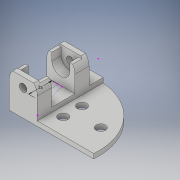
# Autodesk Inventor part: beta_plate
Saved by Autodesk Inventor 2018 (Build 220112000, 112)
## iProperties
Created: 2017-10-04
Part Number: beta_plate
Material: Generic
Document SubType Name: Modeling
Designer: rheal
Density: 1 g/cm^3
Appearance: Default
Author: rheal
Autodesk Inventor part; units mm, degrees
ref_plane "Work Plane12" through (0, 0, 0) normal (0, 1, 0) x (1, 0, 0)
sketch "Sketch2" plane through (0, 0, 0) normal (0, 1, 0) x (1, 0, 0)
  line L0 (-10, -65) -> (-10, -85)
  line L1 (-10, -85) -> (20, -85)
  line L2 (-10, -50) -> (-10, -15)
  line L3 (17.5697, -20.0796) -> (74.4447, -85.0796) construction
  line L4 (80.25, -80) -> (80.25, -36.3042) construction
  line L5 (-10, -65) -> (-10, -50)
  arc A0 (80.25, -80) -> (23.375, -15) centre (15.252, -79.4904) ccw projected
  line L6 (20, -85) -> (20, -15)
  line L7 (20, -85) -> (90, -85) construction
  line L8 (20, -15) -> (-10, -15)
  point P0 (0, -80)
  point P1 (0, 0)
  dimension "d13" = 30
  dimension "d14" = 20
  dimension "d15" = 35
  dimension "d98" = 70
  dimension "d99" = 90
  constraints: 16 end point, 3 vertical, 1 horizontal, 1 perpendicular, 1 other
  measures "d13" distance of L1.end L0.end
  measures "d14" distance of L0.end L0.start
  measures "d15" distance of L2.start L2.end
  measures "d98" distance of L1.end L6.end
  measures "d99" angle of L7 L6
extrude "Extrusion2" add sketch "Sketch2" along normal blind 5
ref_plane "Work Plane7" through (0, 5, 0) normal (0, 1, 0) x (1, 0, 0)
ref_plane "Work Plane6" through (0, 5, 0) normal (0, 1, 0) x (1, 0, 0)
sketch "Sketch7" plane through (0, 5, 0) normal (0, 1, 0) x (1, 0, 0)
  line L0 (-2.5, -32.5) -> (7.5, -32.5) projected
  line L1 (2.5, -32.5) -> (15, -75.625) construction
  line L2 (15, -85) -> (15, -65) projected
  line L3 (-2.5, -45) -> (7.5, -45) projected
  line L4 (2.5, -45) -> (2.5, -70) construction
  line L5 (2.5, -57.5) -> (-13.1217, -57.5) construction
  point P0 (0, 0)
  point P1 (20, -85)
  dimension "d54" = 25
  constraints: 6 end point, 3 midpoint, 1 horizontal, 1 vertical, 2 other
  measures "d54" distance of L4.start L4.end
ref_plane "Work Plane8" through (-2.5, 5, 45) normal (0, 0, 1) x (1, 0, 0)
sketch "Sketch8" plane through (-2.5, 5, 45) normal (0, 0, 1) x (1, 0, 0)
  line L0 (-7.5, 0) -> (22.5, 0) projected
  arc A0 (22.5, 18) -> (-7.5, 18) centre (7.5, 18) ccw
  line L1 (-7.5, 18) -> (-7.5, 0)
  line L2 (22.5, 18) -> (22.5, 0)
  point P0 (2.5, -5)
  dimension "d100" = 30
  constraints: 4 end point, 2 point on circle, 1 centre point, 1 parallel, 1 vertical
  measures "d100" diameter of A0
extrude "Extrusion7" add sketch "Sketch8" against normal blind 15
ref_plane "Work Plane9" through (-2.5, 5, 45) normal (0, 0, 1) x (1, 0, 0)
sketch "Sketch9" plane through (-2.5, 5, 45) normal (0, 0, 1) x (1, 0, 0)
  arc A0 (-2, 18) -> (17, 18) centre (7.5, 18) ccw
  line L0 (-2, 18) -> (-2, 26.124)
  line L1 (17, 18) -> (17, 26.124)
  line L2 (22.5, 0) -> (-7.5, 0) construction
  line L3 (7.5, 0) -> (7.5, 18) construction
  arc A1 (22.5, 18) -> (-7.5, 18) centre (7.5, 18) ccw construction
  line L4 (17, 26.124) -> (20.1095, 26.124)
  line L5 (-2, 26.124) -> (-5.1095, 26.124)
  arc A2 (20.1095, 26.124) -> (-5.1095, 26.124) centre (7.5, 18) ccw
  point P0 (2.5, -5)
  dimension "d47" = 19
  constraints: 10 end point, 6 point on circle, 2 centre point, 1 concentric, 1 horizontal, 1 midpoint, 1 point on line
  measures "d47" diameter of A0
extrude "Extrusion8" cut sketch "Sketch9" against normal blind 10
ref_plane "Work Plane10" through (2.5, 23, 30) normal (0, 0, -1) x (-1, 0, 0)
sketch "Sketch10" plane through (2.5, 23, 30) normal (0, 0, -1) x (-1, 0, 0)
  line L0 (-5, 0) -> (5, 0) projected
  arc A0 (-12, 0) -> (7, 0) centre (-2.5, 0) ccw projected
  circle A1 centre (-2.5, 0) radius 4
  point P0 (2.5, -23)
  dimension "d103" = 8
  constraints: 1 centre point, 1 coincident
  measures "d103" diameter of A1
extrude "Extrusion9" cut sketch "Sketch10" against normal blind 5
ref_plane "Work Plane2" through (2.5, 5, 57.5) normal (0, 0, 1) x (1, 0, 0)
mirror "Mirror2" about plane through (2.5, 5, 57.5) normal (0, 0, 1) of "Extrusion7", "Extrusion8", "Extrusion9"
ref_plane "Work Plane11" through (2.5, 23, 85) normal (0, 0, 1) x (1, 0, 0)
sketch "Sketch11" plane through (2.5, 23, 85) normal (0, 0, 1) x (1, 0, 0)
  line L0 (-12.5, 20) -> (17.5, 20)
  line L1 (17.5, 20) -> (17.5, 10)
  line L2 (17.5, 10) -> (-12.5, 10)
  line L3 (-12.5, 10) -> (-12.5, 20)
  arc A0 (17.5, 0) -> (-12.5, 0) centre (2.5, 0) ccw projected
  line L4 (-12.5, 20) -> (17.5, 10) construction
  line L5 (17.5, 20) -> (-12.5, 10) construction
  point P0 (-2.5, -23)
  point P1 (2.5, 15)
  dimension "d101" = 30
  dimension "d102" = 10
  constraints: 12 end point, 2 midpoint, 2 parallel, 1 horizontal, 1 perpendicular, 1 point on circle
  measures "d101" distance of L1.end L2.end
  measures "d102" distance of L0.end L1.end
extrude "Extrusion10" cut sketch "Sketch11" against normal blind 80
ref_plane "Work Plane14" through (0, 0, 0) normal (0, -1, 0) x (1, 0, 0)
sketch "Sketch17" plane through (0, 0, 0) normal (0, -1, 0) x (1, 0, 0)
  line L0 (15, 15) -> (-10, 15) projected
  line L1 (-10, 15) -> (15, 15)
  line L2 (-10, 15) -> (-10, 30) projected
  line L3 (-10, 15) -> (-10, 85)
  line L4 (-10, 85) -> (80, 85)
  arc A0 (15, 15) -> (80, 85) centre (15, 80.1786) ccw
  point P0 (0, 0)
  dimension "d94" = 90
  constraints: 6 end point, 2 point on circle, 1 centre point, 1 collinear, 1 horizontal, 1 tangent
  measures "d94" distance of L3.end L4.end
extrude "Extrusion16" add sketch "Sketch17" along normal blind 5
sketch "Sketch18" plane through (0, 0, 0) normal (0, 1, 0) x (1, 0, 0)
  line L0 (20, -70) -> (20, -45) construction
  line L1 (20, -57.5) -> (60, -57.5) construction
  line L2 (20, -57.5) -> (30, -57.5) construction
  line L3 (30, -57.5) -> (30, -37.5) construction
  line L4 (30, -57.5) -> (30, -77.5) construction
  circle A0 centre (30, -67.5) radius 5
  circle A1 centre (30, -47.5) radius 5
  circle A2 centre (60, -57.5) radius 5
  point P0 (0, 0)
  dimension "d104" = 40
  dimension "d105" = 10
  dimension "d106" = 20
  dimension "d107" = 20
  dimension "d108" = 10
  dimension "d109" = 10
  dimension "d110" = 10
  constraints: 8 end point, 3 centre point, 3 midpoint, 2 perpendicular, 1 coincident, 1 horizontal, 1 point on line
  measures "d104" distance of L1.start L1.end
  measures "d105" distance of L1.start L2.end
  measures "d106" distance of L2.end L3.end
  measures "d107" distance of L2.end L4.end
  measures "d108" diameter of A0
  measures "d109" diameter of A1
  measures "d110" diameter of A2
extrude "Extrusion17" cut sketch "Sketch18" against normal blind 5
body "Solid1"
